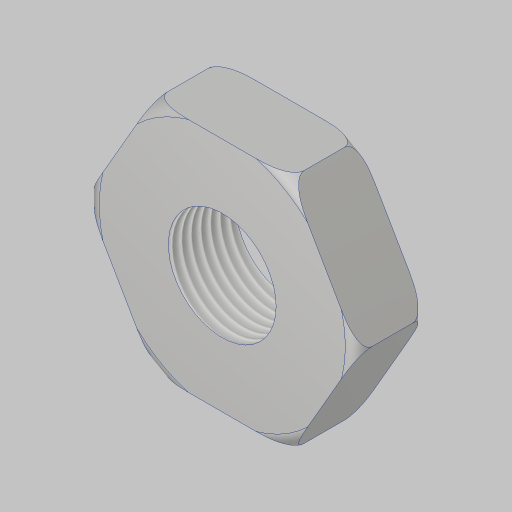
# Autodesk Inventor part: EL2-A-012
Saved by Autodesk Inventor 2023.5 (Build 275446000, 446)
## iProperties
Created: 2025-01-25
Part Number: EL2-A-012
Material: Aluminum 6061
Document SubType Name: Modeling
Designer: brand
Density: 2.7 g/cm^3
Appearance: Aluminum - Flat
Author: brand
Autodesk Inventor part; units mm, degrees
ref_plane "YZ Plane" through (0, 0, 0) normal (1, 0, 0) x (0, 1, 0)
ref_plane "XZ Plane" through (0, 0, 0) normal (0, 1, 0) x (-1, 0, 0)
ref_plane "XY Plane" through (0, 0, 0) normal (0, 0, 1) x (1, 0, 0)
sketch "Sketch1" plane through (0, 0, 0) normal (0, 0, 1) x (1, 0, 0)
  line L0 (25.6632, 0) -> (12.8316, -22.225)
  line L1 (12.8316, -22.225) -> (-12.8316, -22.225)
  line L2 (-12.8316, -22.225) -> (-25.6632, 0)
  line L3 (-25.6632, 0) -> (-12.8316, 22.225)
  line L4 (-12.8316, 22.225) -> (12.8316, 22.225)
  line L5 (12.8316, 22.225) -> (25.6632, 0)
  point P0 (0, 0)
  point P1 (0, 0)
  dimension "d1" = 44.45
  constraints: 12 end point, 1 coincident, 1 horizontal alignment, 13 other
  measures "d1" distance between parallel lines of L1 L4
extrude "Extrusion1" add sketch "Sketch1" along normal mid plane 12.7
sketch "Sketch2" plane through (0, 0, 6.35) normal (0, 0, 1) x (1, 0, 0)
  point P0 (0, 0)
hole "Hole1" at (0, 0, 6.35) direction (0, 0, -1) diameter 20.2692 end through all thread size "7/8-14 UNF" class "2B" standard "ANSI Unified Screw Threads"
sketch "Sketch3" plane through (0, 0, 0) normal (0, 1, 0) x (-1, 0, 0)
  line L0 (-10.1346, 6.35) -> (-10.1346, -6.35) construction
  line L1 (-10.1346, -6.35) -> (-25.6632, -6.35) construction
  line L2 (-25.6632, -6.35) -> (-25.6632, 6.35) construction
  line L3 (-25.6632, 6.35) -> (-10.1346, 6.35) construction
  line L4 (10.1346, -6.35) -> (10.1346, 6.35) construction
  line L5 (10.1346, 6.35) -> (25.6632, 6.35) construction
  line L6 (25.6632, 6.35) -> (25.6632, -6.35) construction
  line L7 (25.6632, -6.35) -> (10.1346, -6.35) construction
  line L8 (-23.1232, 6.35) -> (-25.6632, 6.35)
  line L9 (-25.6632, 6.35) -> (-25.6632, 3.81)
  arc A0 (-23.1232, 6.35) -> (-25.6632, 3.81) centre (-23.1232, 3.81) ccw
  line L10 (-25.6632, 0) -> (-10.1346, 0) construction
  line L11 (-10.1346, -6.35) -> (-10.1346, 6.35) construction
  line L12 (-23.1232, -6.35) -> (-25.6632, -6.35)
  line L13 (-25.6632, -6.35) -> (-25.6632, -3.81)
  arc A1 (-25.6632, -3.81) -> (-23.1232, -6.35) centre (-23.1232, -3.81) ccw
  line L14 (0, -9.8106) -> (0, 9.8106) projected
  point P0 (0, 0)
  dimension "d11" = 2.54
  dimension "d12" = 2.54
  dimension "d13" = 2.54
  constraints: 10 end point, 4 point on circle, 3 symmetric about line, 2 centre point, 2 midpoint, 2 point on line, 1 horizontal, 1 perpendicular, 1 other
  measures "d11" distance of L2.end L9.end
  measures "d12" distance of L2.end L8.start
  measures "d13" radius of A0
revolve "Revolution1" cut sketch "Sketch3" angle 360 about axis through (0, 0, -10) along (0, 0, 1)
equation "\"d12\" = d11"
equation "\"d13\" = d11"
body "Solid1"
